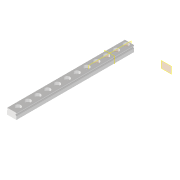
# Autodesk Inventor part: 30_Cube_Z_Focus_MGN_NEMA_rail
Saved by Autodesk Inventor 2022 (Build 260153000, 153)
## iProperties
Created: 2021-05-02
Part Number: 30_Cube_Z_Focus_MGN_NEMA_rail
Material: Generic
Document SubType Name: Modeling
Designer: diederichbenedict
Density: 1 g/cm^3
Appearance: Default
Catalog Web Link: https://3d-druckershop.com/p/mgn12-linearfuehrungsschiene-laenge-300-mm-kaufen
Description: Has to be cut!
Author: diederichbenedict
Autodesk Inventor part; units mm, degrees
ref_plane "YZ Plane" through (0, 0, 0) normal (1, 0, 0) x (0, 1, 0)
ref_plane "XZ Plane" through (0, 0, 0) normal (0, 1, 0) x (-1, 0, 0)
ref_plane "XY Plane" through (0, 0, 0) normal (0, 0, 1) x (1, 0, 0)
ref_plane "Work Plane1" through (0, 0, 0) normal (0, 0, 1) x (1, 0, 0)
sketch "Sketch1" plane through (0, 0, 0) normal (0, 0, 1) x (1, 0, 0)
  line L0 (0, 0) -> (5.55, 0)
  line L1 (6.05, -7.8) -> (0, -7.8)
  line L2 (0, -7.8) -> (0, 0)
  line L3 (5.55, 0) -> (6.05, -0.5)
  arc A0 (6.05, -3.6294) -> (5.8482, -3.4873) centre (5.8013, -3.7683) ccw
  arc A1 (5.5514, -3.0941) -> (5.8482, -3.4873) centre (6.6343, -2.5853) ccw
  arc A2 (5.5514, -3.0941) -> (5.425, -2.9829) centre (5.3332, -3.2146) ccw
  line L4 (5.425, -2.9829) -> (4.928, -2.9441)
  arc A3 (4.7, -2.7255) -> (4.928, -2.9441) centre (4.9475, -2.6956) ccw
  arc A4 (4.9275, -2.0261) -> (4.7, -2.2744) centre (4.9493, -2.2744) ccw
  arc A5 (5.293, -1.9942) -> (5.5514, -1.8412) centre (5.3208, -1.7464) ccw
  arc A6 (5.8954, -1.3233) -> (5.5514, -1.8412) centre (6.7024, -2.2326) ccw
  arc A7 (5.8954, -1.3233) -> (6.05, -1.1) centre (5.8008, -1.0927) ccw
  line L5 (5.293, -1.9942) -> (4.9275, -2.0261)
  line L6 (4.7, -2.7255) -> (4.7, -2.2744)
  line L7 (6.05, -0.5) -> (6.05, -1.1)
  line L8 (6.05, -3.6294) -> (6.05, -7.8)
  point P0 (6.05, 0)
  dimension "d0" = 0.5
  dimension "d1" = 0.5
  dimension "d17" = 6.05
  dimension "d18" = 7.8
  dimension "d20" = 2.6756
  dimension "d21" = 0.5
  dimension "d22" = 1.1
  dimension "d23" = 4.7
  dimension "d24" = 0.2275
  dimension "d25" = 0.228
  dimension "d26" = 0
  dimension "d27" = 0.2483
  dimension "d28" = 0.2186
  constraints: 18 end point, 16 point on circle, 8 centre point, 3 parallel, 2 perpendicular, 1 coincident, 1 horizontal, 1 point on line
  measures "d0" distance of L0.end point (6.05, 0)
  measures "d1" distance of L3.end point (6.05, 0)
  measures "d17" distance between parallel lines of L2 L7
  measures "d18" distance between parallel lines of L1 L0
  measures "d20" distance of A7.centre A0.centre
  measures "d21" distance from line of L3.end L0
  measures "d22" distance from line of L7.end L0
  measures "d23" distance between parallel lines of L6 L2
  measures "d24" horizontal distance of L5.end L6.end
  measures "d25" distance from line of L4.end L6
  measures "d26" horizontal distance of A1.start A5.end
  measures "d27" vertical distance of L5.end L6.end
  measures "d28" vertical distance of L4.end L6.start
extrude "Extrusion1" add sketch "Sketch1" along normal blind 50
mirror "Mirror1" about plane through (0, 0, 0) normal (-1, 0, 0) of "Extrusion1"
sketch "Sketch2" plane through (5.55, 0, 50) normal (0, 1, 0) x (1, 0, 0)
  line L0 (-11.1, 50) -> (0, 50) projected
  line L1 (-11.1, 50) -> (-11.1, 0) projected
  line L2 (0, 0) -> (-11.1, 0) projected
  line L3 (0, 50) -> (0, 0) projected
  point P0 (-5.55, 50)
  point P1 (-5.45, 45.5983)
hole "Hole1" at (0.1, 0, 4.4017) direction (0, -1, 0) diameter 3.5 end through all counterbore diameter 7 counterbore depth 3.5
pattern_linear "Rectangular Pattern1" count 5 spacing 12.5 along (0, 0, 1) of "Hole1"
ref_plane "Work Plane2" through (0, -7.8, 0) normal (1, 0, 0) x (0, 0, -1)
ref_plane "Arbeitsebene3" through (0, 0, 25) normal (0, 0, 1) x (1, 0, 0)
pattern_linear "Rechteckige Anordnung2" count 3 spacing 50 along (0, 0, 1) of "Extrusion1", "Mirror1", "Hole1", "Rectangular Pattern1"
ref_plane "Arbeitsebene4" through (0, 0, 75) normal (0, 0, -1) x (-1, 0, 0)
ref_plane "Arbeitsebene5" through (0, -7.8, 0) normal (-1, 0, 0) x (0, 0, 1)
equation "\"d1\" = d0"
body "Solid1"
